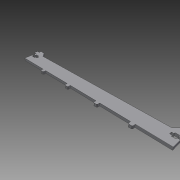
# Autodesk Inventor part: frame_brace_top
Saved by Autodesk Inventor 2014 (Build 180170000, 170)
## iProperties
Created: 2013-12-06
Part Number: frame_brace_top
Material: Generic
Document SubType Name: Modeling
Designer: buben
Density: 1 g/cm^3
Appearance: Default
Author: buben
Autodesk Inventor part; units mm, degrees
ref_plane "YZ Plane" through (0, 0, 0) normal (1, 0, 0) x (0, 1, 0)
ref_plane "XZ Plane" through (0, 0, 0) normal (0, 1, 0) x (-1, 0, 0)
ref_plane "XY Plane" through (0, 0, 0) normal (0, 0, 1) x (1, 0, 0)
sketch "Sketch1" plane through (0, 0, 0) normal (0, 0, 1) x (1, 0, 0)
  line L0 (0, 0) -> (335, 0)
  line L1 (335, 0) -> (335, 40)
  line L2 (0, 40) -> (0, 0)
  line L3 (10, 40) -> (20, 30)
  line L4 (20, 30) -> (315, 30)
  line L5 (315, 30) -> (325, 40)
  line L6 (335, 40) -> (325, 40)
  line L7 (10, 40) -> (0, 40)
  dimension "d0" = 335
  dimension "d1" = 40
  dimension "d2" = 45
  dimension "d3" = 10
  dimension "d4" = 10
  dimension "d5" = 10
  constraints: 16 end point, 3 parallel, 3 perpendicular, 1 collinear, 1 horizontal
  measures "d0" distance of L0.start L0.end
  measures "d1" distance of L2.start L0.start
  measures "d2" angle of L7 L3
  measures "d3" distance of L3.start L2.start
  measures "d4" distance between parallel lines of L7 L4
  measures "d5" distance of L1.end L5.end
extrude "Extrusion1" add sketch "Sketch1" along normal blind 6
sketch "Sketch2" plane through (0, 0, 6) normal (0, 0, 1) x (1, 0, 0)
  line L0 (0, 0) -> (335, 0) projected
  line L1 (315, 30) -> (20, 30) projected
  line L2 (0, 40) -> (0, 0) projected
  line L3 (0, 17.75) -> (0, 22.25)
  line L4 (16.3, 22.25) -> (16.3, 17.75)
  line L5 (5, 24.75) -> (12.3, 24.75)
  line L6 (12.3, 15.25) -> (5, 15.25)
  line L7 (0, 22.25) -> (5, 22.25)
  line L8 (12.3, 22.25) -> (16.3, 22.25)
  line L9 (16.3, 17.75) -> (12.3, 17.75)
  line L10 (5, 17.75) -> (0, 17.75)
  line L11 (5, 15.25) -> (5, 17.75)
  line L12 (5, 22.25) -> (5, 24.75)
  line L13 (12.3, 24.75) -> (12.3, 22.25)
  line L14 (12.3, 17.75) -> (12.3, 15.25)
  line L15 (167.5, 0) -> (167.5, 30) construction
  line L16 (335, 17.75) -> (335, 22.25)
  line L17 (318.7, 22.25) -> (318.7, 17.75)
  line L18 (330, 24.75) -> (322.7, 24.75)
  line L19 (322.7, 15.25) -> (330, 15.25)
  line L20 (335, 22.25) -> (330, 22.25)
  line L21 (322.7, 22.25) -> (318.7, 22.25)
  line L22 (318.7, 17.75) -> (322.7, 17.75)
  line L23 (330, 17.75) -> (335, 17.75)
  line L24 (330, 15.25) -> (330, 17.75)
  line L25 (330, 22.25) -> (330, 24.75)
  line L26 (322.7, 24.75) -> (322.7, 22.25)
  line L27 (322.7, 17.75) -> (322.7, 15.25)
  point P0 (0, 20)
  point P1 (0, 20)
  point P2 (335, 20)
  point P3 (335, 20)
  dimension "d8" = 4.5
  dimension "d9" = 2.5
  dimension "d10" = 2.5
  dimension "d11" = 5
  dimension "d12" = 7.3
  dimension "d13" = 4
  constraints: 50 end point, 14 symmetric about line, 10 parallel, 5 collinear, 4 midpoint, 4 perpendicular, 3 horizontal, 1 coincident
  measures "d8" distance of L4.start L4.end
  measures "d9" distance of L5.end L8.start
  measures "d10" distance of L9.end L6.start
  measures "d11" distance of L10.start L3.start
  measures "d12" distance of L6.start L6.end
  measures "d13" distance of L4.end L9.end
extrude "Extrusion2" cut sketch "Sketch2" against normal blind 6
sketch "Sketch3" plane through (0, 0, 6) normal (0, 0, 1) x (1, 0, 0)
  line L0 (0, 17.75) -> (0, 0) projected
  line L1 (0, 0) -> (335, 0) projected
  line L2 (335, 0) -> (335, 17.75) projected
  line L3 (335, 22.25) -> (335, 40) projected
  line L4 (0, 40) -> (0, 22.25) projected
  line L5 (16.3, 22.25) -> (16.3, 17.75) projected
  line L6 (0, 35.5) -> (-4, 35.5)
  line L7 (-6, 33.5) -> (-6, 29.5)
  line L8 (-4, 27.5) -> (0, 27.5)
  line L9 (0, 27.5) -> (0, 35.5)
  line L10 (0, 12.5) -> (-4, 12.5)
  line L11 (-6, 10.5) -> (-6, 6.5)
  line L12 (-4, 4.5) -> (0, 4.5)
  line L13 (0, 4.5) -> (0, 12.5)
  arc A0 (-4, 35.5) -> (-6, 33.5) centre (-4, 33.5) ccw
  arc A1 (-6, 29.5) -> (-4, 27.5) centre (-4, 29.5) ccw
  arc A2 (-4, 12.5) -> (-6, 10.5) centre (-4, 10.5) ccw
  arc A3 (-6, 6.5) -> (-4, 4.5) centre (-4, 6.5) ccw
  line L14 (335, 35.5) -> (339, 35.5)
  line L15 (341, 33.5) -> (341, 29.5)
  line L16 (339, 27.5) -> (335, 27.5)
  line L17 (335, 27.5) -> (335, 35.5)
  line L18 (335, 12.5) -> (339, 12.5)
  line L19 (341, 10.5) -> (341, 6.5)
  line L20 (339, 4.5) -> (335, 4.5)
  line L21 (335, 4.5) -> (335, 12.5)
  arc A4 (341, 33.5) -> (339, 35.5) centre (339, 33.5) ccw
  arc A5 (339, 27.5) -> (341, 29.5) centre (339, 29.5) ccw
  arc A6 (341, 10.5) -> (339, 12.5) centre (339, 10.5) ccw
  arc A7 (339, 4.5) -> (341, 6.5) centre (339, 6.5) ccw
  line L22 (197.8, 0) -> (205.8, 0)
  line L23 (205.8, 0) -> (205.8, -4)
  line L24 (203.8, -6) -> (199.8, -6)
  line L25 (197.8, -4) -> (197.8, 0)
  line L26 (137.2, 0) -> (129.2, 0)
  line L27 (129.2, 0) -> (129.2, -4)
  line L28 (131.2, -6) -> (135.2, -6)
  line L29 (137.2, -4) -> (137.2, 0)
  line L30 (60.6, 0) -> (68.6, 0)
  line L31 (68.6, 0) -> (68.6, -4)
  line L32 (66.6, -6) -> (62.6, -6)
  line L33 (60.6, -4) -> (60.6, 0)
  line L34 (266.4, 0) -> (274.4, 0)
  line L35 (274.4, 0) -> (274.4, -4)
  line L36 (272.4, -6) -> (268.4, -6)
  line L37 (266.4, -4) -> (266.4, 0)
  arc A8 (60.6, -4) -> (62.6, -6) centre (62.6, -4) ccw
  arc A9 (66.6, -6) -> (68.6, -4) centre (66.6, -4) ccw
  arc A10 (129.2, -4) -> (131.2, -6) centre (131.2, -4) ccw
  arc A11 (135.2, -6) -> (137.2, -4) centre (135.2, -4) ccw
  arc A12 (197.8, -4) -> (199.8, -6) centre (199.8, -4) ccw
  arc A13 (203.8, -6) -> (205.8, -4) centre (203.8, -4) ccw
  arc A14 (266.4, -4) -> (268.4, -6) centre (268.4, -4) ccw
  arc A15 (272.4, -6) -> (274.4, -4) centre (272.4, -4) ccw
  line L38 (68.6, -2) -> (129.2, -2) construction
  line L39 (137.2, -2) -> (197.8, -2) construction
  line L40 (205.8, -2) -> (266.4, -2) construction
  line L41 (274.4, -2) -> (335, -2) construction
  line L42 (60.6, -2) -> (0, -2) construction
  point P0 (16.3, 20)
  point P1 (167.5, 0)
  dimension "d16" = 2
  dimension "d17" = 8
  dimension "d18" = 8
  dimension "d19" = 15
  dimension "d20" = 7.5
  dimension "d21" = 6
  dimension "d22" = 2
  dimension "d23" = 6
  dimension "d24" = 2
  dimension "d25" = 8
  dimension "d26" = 8
  dimension "d27" = 8
  dimension "d28" = 8
  dimension "d29" = 6
  constraints: 74 end point, 32 point on circle, 32 tangent, 16 centre point, 16 parallel, 15 collinear, 13 equal radius, 10 midpoint, 8 horizontal, 8 perpendicular, 8 point on line, 2 vertical alignment
  measures "d16" radius of A0
  measures "d17" distance between parallel lines of L12 L10
  measures "d18" distance between parallel lines of L6 L8
  measures "d19" distance between parallel lines of L10 L8
  measures "d20" distance from line of point (16.3, 20) L8
  measures "d21" distance between parallel lines of L4 L7
  measures "d22" radius of A4
  measures "d23" distance between parallel lines of L3 L15
  measures "d24" radius of A8
  measures "d25" distance between parallel lines of L31 L33
  measures "d26" distance between parallel lines of L29 L27
  measures "d27" distance between parallel lines of L23 L25
  measures "d28" distance between parallel lines of L35 L37
  measures "d29" distance between parallel lines of L1 L32
extrude "Extrusion3" add sketch "Sketch3" against normal blind 6
sketch "Sketch4" plane through (0, 0, 6) normal (0, 0, 1) x (1, 0, 0)
  line L0 (0, 12.5) -> (-4, 12.5) projected
  arc A0 (-4, 12.5) -> (-6, 10.5) centre (-4, 10.5) ccw projected
  line L1 (-6, 10.5) -> (-6, 6.5) projected
  arc A1 (-6, 6.5) -> (-4, 4.5) centre (-4, 6.5) ccw projected
  line L2 (-4, 4.5) -> (0, 4.5) projected
  line L3 (335, 4.5) -> (339, 4.5) projected
  arc A2 (339, 4.5) -> (341, 6.5) centre (339, 6.5) ccw projected
  line L4 (341, 6.5) -> (341, 10.5) projected
  arc A3 (341, 10.5) -> (339, 12.5) centre (339, 10.5) ccw projected
  line L5 (339, 12.5) -> (335, 12.5) projected
  line L6 (5, 15.25) -> (5, 17.75) projected
  line L7 (0, 12.5) -> (0, 4.5)
  line L8 (335, 12.5) -> (335, 4.5)
  constraints: 4 end point, 2 parallel
extrude "Extrusion4" cut sketch "Sketch4" against normal blind 6
body "Solid1"
